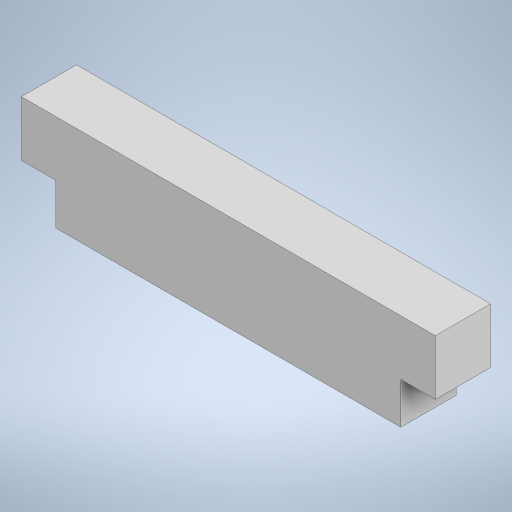
# Autodesk Inventor part: Aletas plato base
Saved by Autodesk Inventor 2023 (Build 270158000, 158)
## iProperties
Created: 2023-11-09
Part Number: Aletas plato base
Material: Genérico
Document SubType Name: Modeling
Designer: JULIAN
Density: 1 g/cm^3
Appearance: Valor por defecto
Author: JULIAN
Autodesk Inventor part; units mm, degrees
ref_plane "YZ Plane" through (0, 0, 0) normal (1, 0, 0) x (0, 1, 0)
ref_plane "XZ Plane" through (0, 0, 0) normal (0, 1, 0) x (-1, 0, 0)
ref_plane "XY Plane" through (0, 0, 0) normal (0, 0, 1) x (1, 0, 0)
sketch "Boceto1" plane through (0, 0, 0) normal (0, 0, 1) x (1, 0, 0)
  line L0 (0, 0) -> (25, 0)
  line L1 (25, 0) -> (25, 3)
  line L2 (25, 3) -> (27.5, 3)
  line L3 (27.5, 3) -> (27.5, 7)
  line L4 (27.5, 7) -> (-2.5, 7)
  line L5 (-2.5, 7) -> (-2.5, 3)
  line L6 (-2.5, 3) -> (0, 3)
  line L7 (0, 3) -> (0, 0)
  dimension "d0" = 25
  dimension "d1" = 3
  dimension "d2" = 2.5
  dimension "d3" = 4
  dimension "d4" = 30
  constraints: 16 end point, 5 perpendicular, 2 point on line, 1 horizontal, 1 vertical
  measures "d0" distance of L0.start L0.end
  measures "d1" distance of L0.end L1.end
  measures "d2" distance of L1.end L2.end
  measures "d3" distance of L2.end L3.end
  measures "d4" distance of L3.end L4.end
extrude "Extrusión1" add sketch "Boceto1" along normal blind 4
